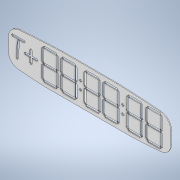
# Autodesk Inventor part: 7 Segment Clock
Saved by Autodesk Inventor 2021 (Build 250183000, 183)
## iProperties
Created: 2020-06-26
Part Number: 7 Segment Clock
Material: White
Document SubType Name: Modeling
Designer: dech3
Density: 1.188 g/cm^3
Appearance: Polycarbonate - Clear
Author: dech3
Autodesk Inventor part; units mm, degrees
(part 1 of 2)
ref_plane "YZ Plane" through (0, 0, 0) normal (1, 0, 0) x (0, 1, 0)
ref_plane "XZ Plane" through (0, 0, 0) normal (0, 1, 0) x (-1, 0, 0)
ref_plane "XY Plane" through (0, 0, 0) normal (0, 0, 1) x (1, 0, 0)
sketch "Single Segment" plane through (0, 0, 0) normal (0, 0, 1) x (1, 0, 0)
  arc A0 (130.9839, -3.9071) -> (131.691, -4.2) centre (131.691, -3.2) ccw
  arc A1 (131.691, 3.8) -> (130.9839, 3.5071) centre (131.691, 2.8) ccw
  line L0 (130.9839, -3.9071) -> (128.0768, -1)
  line L1 (130.9839, 3.5071) -> (128.0768, 0.6)
  line L2 (128.0768, -0.2) -> (128.0768, -1)
  line L3 (128.0768, -0.2) -> (128.0768, 0.6)
  line L4 (131.691, 3.8) -> (174.4626, 3.8)
  line L5 (174.4626, -4.2) -> (131.691, -4.2)
  arc A2 (175.1697, 3.5071) -> (174.4626, 3.8) centre (174.4626, 2.8) ccw
  line L6 (175.1697, 3.5071) -> (178.0768, 0.6)
  line L7 (178.0768, -0.2) -> (178.0768, 0.6)
  line L8 (178.0768, -0.2) -> (178.0768, -1)
  arc A3 (174.4626, -4.2) -> (175.1697, -3.9071) centre (174.4626, -3.2) ccw
  line L9 (175.1697, -3.9071) -> (178.0768, -1)
  point P0 (153.0768, 0)
  point P1 (131.2768, -4.2)
  point P2 (131.2768, 3.8)
  point P3 (174.8768, 3.8)
  point P4 (174.8768, -4.2)
  dimension "d105" = 3.2
  dimension "d108" = 3.2
  dimension "d111" = 3.2
  dimension "d112" = 3.2
  dimension "d113" = 3.2
  dimension "d114" = 3.2
  dimension "d115" = 3.2
  dimension "d116" = 1
  dimension "d117" = 8
  dimension "d118" = 8
  dimension "d121" = 3.2
  dimension "d122" = 3.2
  dimension "d123" = 50
  dimension "d126" = 135
  dimension "d127" = 50
  dimension "d128" = 135
  dimension "d129" = 4
  dimension "d130" = 4
  measures "d105" horizontal distance of point (131.277, -4.2) L0.end
  measures "d108" horizontal distance of L7.end point (174.877, 3.8)
  measures "d111" horizontal distance of point (131.277, 3.8) L3.end
  measures "d112" horizontal distance of L9.end point (174.877, -4.2)
  measures "d113" horizontal distance of L9.end point (174.877, -4.2)
  measures "d114" horizontal distance of point (131.277, 3.8) L3.end
  measures "d115" horizontal distance of point (131.277, -4.2) L0.end
  measures "d116" radius of A1
  measures "d117" distance of point (174.877, -4.2) point (174.877, 3.8)
  measures "d118" distance of point (131.277, -4.2) point (131.277, 3.8)
  measures "d121" horizontal distance of L7.end point (174.877, 3.8)
  measures "d122" horizontal distance of point (174.877, -4.2) L8.start
  measures "d123" distance of L8.start L3.start
  measures "d126" angle of L5 L9
  measures "d127" horizontal distance of L9.end L3.start
  measures "d128" angle of L4 L6
  measures "d129" vertical distance of L8.start point (174.877, -4.2)
  measures "d130" vertical distance of point (131.277, -4.2) L3.start
sketch "7 Segment Digit" plane through (0, 0, 0) normal (0, 0, 1) x (1, 0, 0)
  arc A0 (217.9071, 45.0929) -> (218.6142, 44.8) centre (218.6142, 45.8) ccw
  arc A1 (218.6142, 52.8) -> (217.9071, 52.5071) centre (218.6142, 51.8) ccw
  line L0 (217.9071, 45.0929) -> (215, 48)
  line L1 (217.9071, 52.5071) -> (215, 49.6)
  line L2 (215, 48.8) -> (215, 48)
  line L3 (215, 48.8) -> (215, 49.6)
  line L4 (218.6142, 52.8) -> (261.3858, 52.8)
  line L5 (261.3858, 44.8) -> (218.6142, 44.8)
  arc A2 (262.0929, 52.5071) -> (261.3858, 52.8) centre (261.3858, 51.8) ccw
  line L6 (262.0929, 52.5071) -> (265, 49.6)
  line L7 (265, 48.8) -> (265, 49.6)
  line L8 (265, 48.8) -> (265, 48)
  arc A3 (261.3858, 44.8) -> (262.0929, 45.0929) centre (261.3858, 45.8) ccw
  line L9 (262.0929, 45.0929) -> (265, 48)
  arc A4 (217.9071, -8.7071) -> (218.6142, -9) centre (218.6142, -8) ccw
  arc A5 (218.6142, -1) -> (217.9071, -1.2929) centre (218.6142, -2) ccw
  line L10 (217.9071, -8.7071) -> (215, -5.8)
  line L11 (217.9071, -1.2929) -> (215, -4.2)
  line L12 (215, -5) -> (215, -5.8)
  line L13 (215, -5) -> (215, -4.2)
  line L14 (218.6142, -1) -> (261.3858, -1)
  line L15 (261.3858, -9) -> (218.6142, -9)
  arc A6 (262.0929, -1.2929) -> (261.3858, -1) centre (261.3858, -2) ccw
  line L16 (262.0929, -1.2929) -> (265, -4.2)
  line L17 (265, -5) -> (265, -4.2)
  line L18 (265, -5) -> (265, -5.8)
  arc A7 (261.3858, -9) -> (262.0929, -8.7071) centre (261.3858, -8) ccw
  line L19 (262.0929, -8.7071) -> (265, -5.8)
  arc A8 (216.8071, -0.1929) -> (217.1, 0.5142) centre (216.1, 0.5142) ccw
  arc A9 (209.1, 0.5142) -> (209.3929, -0.1929) centre (210.1, 0.5142) ccw
  line L20 (216.8071, -0.1929) -> (213.9, -3.1)
  line L21 (209.3929, -0.1929) -> (212.3, -3.1)
  line L22 (213.1, -3.1) -> (213.9, -3.1)
  line L23 (213.1, -3.1) -> (212.3, -3.1)
  line L24 (209.1, 0.5142) -> (209.1, 43.2858)
  line L25 (217.1, 43.2858) -> (217.1, 0.5142)
  arc A10 (209.3929, 43.9929) -> (209.1, 43.2858) centre (210.1, 43.2858) ccw
  line L26 (209.3929, 43.9929) -> (212.3, 46.9)
  line L27 (213.1, 46.9) -> (212.3, 46.9)
  line L28 (213.1, 46.9) -> (213.9, 46.9)
  arc A11 (217.1, 43.2858) -> (216.8071, 43.9929) centre (216.1, 43.2858) ccw
  line L29 (216.8071, 43.9929) -> (213.9, 46.9)
  arc A12 (216.8071, -53.9929) -> (217.1, -53.2858) centre (216.1, -53.2858) ccw
  arc A13 (209.1, -53.2858) -> (209.3929, -53.9929) centre (210.1, -53.2858) ccw
  line L30 (216.8071, -53.9929) -> (213.9, -56.9)
  line L31 (209.3929, -53.9929) -> (212.3, -56.9)
  line L32 (213.1, -56.9) -> (213.9, -56.9)
  line L33 (213.1, -56.9) -> (212.3, -56.9)
  line L34 (209.1, -53.2858) -> (209.1, -10.5142)
  line L35 (217.1, -10.5142) -> (217.1, -53.2858)
  arc A14 (209.3929, -9.8071) -> (209.1, -10.5142) centre (210.1, -10.5142) ccw
  line L36 (209.3929, -9.8071) -> (212.3, -6.9)
  line L37 (213.1, -6.9) -> (212.3, -6.9)
  line L38 (213.1, -6.9) -> (213.9, -6.9)
  arc A15 (217.1, -10.5142) -> (216.8071, -9.8071) centre (216.1, -10.5142) ccw
  line L39 (216.8071, -9.8071) -> (213.9, -6.9)
  arc A16 (270.6071, -0.1929) -> (270.9, 0.5142) centre (269.9, 0.5142) ccw
  arc A17 (262.9, 0.5142) -> (263.1929, -0.1929) centre (263.9, 0.5142) ccw
  line L40 (270.6071, -0.1929) -> (267.7, -3.1)
  line L41 (263.1929, -0.1929) -> (266.1, -3.1)
  line L42 (266.9, -3.1) -> (267.7, -3.1)
  line L43 (266.9, -3.1) -> (266.1, -3.1)
  line L44 (262.9, 0.5142) -> (262.9, 43.2858)
  line L45 (270.9, 43.2858) -> (270.9, 0.5142)
  arc A18 (263.1929, 43.9929) -> (262.9, 43.2858) centre (263.9, 43.2858) ccw
  line L46 (263.1929, 43.9929) -> (266.1, 46.9)
  line L47 (266.9, 46.9) -> (266.1, 46.9)
  line L48 (266.9, 46.9) -> (267.7, 46.9)
  arc A19 (270.9, 43.2858) -> (270.6071, 43.9929) centre (269.9, 43.2858) ccw
  line L49 (270.6071, 43.9929) -> (267.7, 46.9)
  arc A20 (270.6071, -53.9929) -> (270.9, -53.2858) centre (269.9, -53.2858) ccw
  arc A21 (262.9, -53.2858) -> (263.1929, -53.9929) centre (263.9, -53.2858) ccw
  line L50 (270.6071, -53.9929) -> (267.7, -56.9)
  line L51 (263.1929, -53.9929) -> (266.1, -56.9)
  line L52 (266.9, -56.9) -> (267.7, -56.9)
  line L53 (266.9, -56.9) -> (266.1, -56.9)
  line L54 (262.9, -53.2858) -> (262.9, -10.5142)
  line L55 (270.9, -10.5142) -> (270.9, -53.2858)
  arc A22 (263.1929, -9.8071) -> (262.9, -10.5142) centre (263.9, -10.5142) ccw
  line L56 (263.1929, -9.8071) -> (266.1, -6.9)
  line L57 (266.9, -6.9) -> (266.1, -6.9)
  line L58 (266.9, -6.9) -> (267.7, -6.9)
  arc A23 (270.9, -10.5142) -> (270.6071, -9.8071) centre (269.9, -10.5142) ccw
  line L59 (270.6071, -9.8071) -> (267.7, -6.9)
  arc A24 (217.9071, -62.5071) -> (218.6142, -62.8) centre (218.6142, -61.8) ccw
  arc A25 (218.6142, -54.8) -> (217.9071, -55.0929) centre (218.6142, -55.8) ccw
  line L60 (217.9071, -62.5071) -> (215, -59.6)
  line L61 (217.9071, -55.0929) -> (215, -58)
  line L62 (215, -58.8) -> (215, -59.6)
  line L63 (215, -58.8) -> (215, -58)
  line L64 (218.6142, -54.8) -> (261.3858, -54.8)
  line L65 (261.3858, -62.8) -> (218.6142, -62.8)
  arc A26 (262.0929, -55.0929) -> (261.3858, -54.8) centre (261.3858, -55.8) ccw
  line L66 (262.0929, -55.0929) -> (265, -58)
  line L67 (265, -58.8) -> (265, -58)
  line L68 (265, -58.8) -> (265, -59.6)
  arc A27 (261.3858, -62.8) -> (262.0929, -62.5071) centre (261.3858, -61.8) ccw
  line L69 (262.0929, -62.5071) -> (265, -59.6)
  point P0 (239.8857, -4.9143)
  dimension "d131" = 1.1
  dimension "d132" = 1.1
  dimension "d137" = 1.1
  dimension "d138" = 1.1
  dimension "d139" = 1.1
  dimension "d140" = 1.1
  dimension "d141" = 1.1
  dimension "d142" = 1.1
  dimension "d143" = 1.1
  dimension "d144" = 1.1
  dimension "d145" = 1.1
  dimension "d146" = 1.1
  dimension "d150" = 1.1
  dimension "d151" = 1.1
  dimension "d152" = 1.1
  dimension "d153" = 1.1
sketch "Slanted Segment Large" plane through (0, 0, 0) normal (0, 0, 1) x (1, 0, 0)
  line L0 (-252.8296, -124.6537) -> (-254.4296, -124.6537)
  line L1 (-254.4296, -124.6537) -> (-257.6296, -127.8537)
  line L2 (-257.6296, -127.8537) -> (-261.6917, -184.8537)
  line L3 (-253.6917, -184.8537) -> (-249.6296, -127.8537)
  line L4 (-249.6296, -127.8537) -> (-252.8296, -124.6537)
  line L5 (-261.6917, -184.8537) -> (-258.4917, -188.0537)
  line L6 (-258.4917, -188.0537) -> (-256.8917, -188.0537)
  line L7 (-256.8917, -188.0537) -> (-253.6917, -184.8537)
  point P0 (-253.3255, -154.094)
  point P1 (-253.6296, -124.6537)
  dimension "d294" = 3.2
  dimension "d295" = 3.2
  dimension "d296" = 8
  dimension "d297" = 3.2
  dimension "d298" = 3.2
  dimension "d299" = 57
  dimension "d304" = 3.2
  dimension "d305" = 3.2
  dimension "d306" = 3.2
  dimension "d307" = 3.2
  measures "d294" horizontal distance of L0.end L1.end
  measures "d295" horizontal distance of L3.end L0.start
  measures "d296" distance of L3.end L1.end
  measures "d297" horizontal distance of L3.end L0.start
  measures "d298" horizontal distance of L0.end L1.end
  measures "d299" vertical distance of L3.end L3.start
  measures "d304" horizontal distance of L5.end L2.end
  measures "d305" horizontal distance of L3.start L6.end
  measures "d306" horizontal distance of L2.end L5.end
  measures "d307" horizontal distance of L3.start L6.end
sketch "+ sign" plane through (0, 0, 0) normal (0, 0, 1) x (1, 0, 0)
  line L0 (-226.2607, 18.0992) -> (-229.1679, 15.1921)
  line L1 (-229.4607, 14.485) -> (-229.4607, -2.7008)
  line L2 (-246.6465, -2.7008) -> (-229.4607, -2.7008)
  line L3 (-247.3536, -2.9937) -> (-250.2607, -5.9008)
  line L4 (-250.2607, -5.9008) -> (-250.2607, -7.5008)
  line L5 (-246.6465, -10.7008) -> (-229.4607, -10.7008)
  line L6 (-229.4607, -10.7008) -> (-229.4607, -27.8865)
  line L7 (-226.2607, -31.5008) -> (-224.6607, -31.5008)
  line L8 (-224.6607, -31.5008) -> (-221.7536, -28.5937)
  line L9 (-221.4607, -27.8865) -> (-221.4607, -10.7008)
  line L10 (-204.275, -2.7008) -> (-221.4607, -2.7008)
  line L11 (-204.275, -10.7008) -> (-221.4607, -10.7008)
  line L12 (-203.5679, -2.9937) -> (-200.6607, -5.9008)
  line L13 (-200.6607, -5.9008) -> (-200.6607, -7.5008)
  line L14 (-247.3536, -10.4079) -> (-250.2607, -7.5008)
  line L15 (-229.1679, -28.5937) -> (-226.2607, -31.5008)
  line L16 (-203.5679, -10.4079) -> (-200.6607, -7.5008)
  line L17 (-221.4607, -2.7008) -> (-221.4607, 14.485)
  line L18 (-221.7536, 15.1921) -> (-224.6607, 18.0992)
  line L19 (-224.6607, 18.0992) -> (-226.2607, 18.0992)
  arc A0 (-229.1679, 15.1921) -> (-229.4607, 14.485) centre (-228.4607, 14.485) ccw
  arc A1 (-221.4607, 14.485) -> (-221.7536, 15.1921) centre (-222.4607, 14.485) ccw
  arc A2 (-203.5679, -2.9937) -> (-204.275, -2.7008) centre (-204.275, -3.7008) ccw
  arc A3 (-204.275, -10.7008) -> (-203.5679, -10.4079) centre (-204.275, -9.7008) ccw
  arc A4 (-229.4607, -27.8865) -> (-229.1679, -28.5937) centre (-228.4607, -27.8865) ccw
  arc A5 (-221.7536, -28.5937) -> (-221.4607, -27.8865) centre (-222.4607, -27.8865) ccw
  arc A6 (-247.3536, -10.4079) -> (-246.6465, -10.7008) centre (-246.6465, -9.7008) ccw
  arc A7 (-246.6465, -2.7008) -> (-247.3536, -2.9937) centre (-246.6465, -3.7008) ccw
  point P0 (-225.4266, -6.7349)
  point P1 (-229.4607, 14.8992)
  point P2 (-247.0607, -2.7008)
  point P3 (-247.0607, -10.7008)
  point P4 (-229.4607, -28.3008)
  point P5 (-221.4607, -28.3008)
  point P6 (-203.8607, -2.7008)
  point P7 (-203.8607, -10.7008)
  point P8 (-221.4607, 14.8992)
  dimension "d259" = 3.2
  dimension "d260" = 3.2
  dimension "d261" = 3.2
  dimension "d262" = 3.2
  dimension "d263" = 3.2
  dimension "d264" = 3.2
  dimension "d265" = 3.2
  dimension "d266" = 3.2
  dimension "d267" = 3.2
  dimension "d268" = 3.2
  dimension "d269" = 3.2
  dimension "d270" = 3.2
  dimension "d271" = 3.2
  dimension "d272" = 0
  dimension "d273" = 0
  dimension "d274" = 8
  dimension "d275" = 8
  dimension "d276" = 0
  dimension "d277" = 0
  dimension "d278" = 3.2
  dimension "d279" = 3.2
  dimension "d280" = 3.2
  dimension "d281" = 90
  dimension "d284" = 17.6
  dimension "d285" = 17.6
  dimension "d286" = 17.6
  dimension "d287" = 17.6
  dimension "d288" = 17.6
  dimension "d289" = 0
  dimension "d290" = 17.6
  dimension "d292" = 1
  dimension "d293" = 1
  measures "d259" distance from line of point (-247.061, -2.701) L4
  measures "d260" horizontal distance of point (-247.061, -2.701) L3.end
  measures "d261" horizontal distance of point (-247.061, -10.701) L14.end
  measures "d262" horizontal distance of point (-247.061, -10.701) L14.end
  measures "d263" horizontal distance of L15.end point (-229.461, -28.301)
  measures "d264" horizontal distance of point (-229.461, -28.301) L15.end
  measures "d265" horizontal distance of point (-221.461, -28.301) L7.end
  measures "d266" horizontal distance of L7.end point (-221.461, -28.301)
  measures "d267" horizontal distance of L16.end point (-203.861, -10.701)
  measures "d268" horizontal distance of point (-203.861, -10.701) L16.end
  measures "d269" horizontal distance of point (-203.861, -2.701) L12.end
  measures "d270" horizontal distance of point (-203.861, -2.701) L12.end
  measures "d271" horizontal distance of L18.end point (-221.461, 14.899)
  measures "d272" distance between parallel lines of L17 L9
  measures "d273" distance between parallel lines of L1 L6
  measures "d274" distance between parallel lines of L17 L1
  measures "d275" distance between parallel lines of L5 L2
  measures "d276" distance between parallel lines of L2 L10
  measures "d277" distance between parallel lines of L5 L11
  measures "d278" horizontal distance of L19.end point (-229.461, 14.899)
  measures "d279" horizontal distance of L19.end point (-229.461, 14.899)
  measures "d280" horizontal distance of L18.end point (-221.461, 14.899)
  measures "d281" angle of L10 L17
  measures "d284" distance of L1.end point (-247.061, -2.701)
  measures "d285" distance of point (-203.861, -2.701) L17.start
  measures "d286" distance of point (-221.461, 14.899) L17.start
  measures "d287" distance of point (-221.461, -28.301) L9.end
  measures "d288" distance of point (-229.461, -28.301) L5.end
  measures "d289" distance of L9.end L11.end
  measures "d290" distance of L9.end point (-203.861, -10.701)
  measures "d292" radius of A0
  measures "d293" radius of A4
sketch "Dot" plane through (0, 0, 0) normal (0, 0, 1) x (1, 0, 0)
  line L0 (-34.9663, 29.5091) -> (-32.9663, 29.5091)
  line L1 (-32.9663, 29.5091) -> (-29.7663, 26.3091)
  line L2 (-29.7663, 26.3091) -> (-29.7663, 24.3091)
  line L3 (-29.7663, 24.3091) -> (-32.9663, 21.1091)
  line L4 (-32.9663, 21.1091) -> (-34.9663, 21.1091)
  line L5 (-34.9663, 21.1091) -> (-38.1663, 24.3091)
  line L6 (-38.1663, 24.3091) -> (-38.1663, 26.3091)
  line L7 (-38.1663, 26.3091) -> (-34.9663, 29.5091)
  point P0 (-33.9663, 25.3091)
  dimension "d311" = 3.2
  dimension "d312" = 3.2
  dimension "d314" = 3.2
  dimension "d315" = 3.2
  dimension "d316" = 3.2
  dimension "d317" = 3.2
  dimension "d318" = 3.2
  dimension "d319" = 3.2
  dimension "d320" = 2
  dimension "d321" = 2
  dimension "d322" = 2
  dimension "d323" = 2
  measures "d311" horizontal distance of L1.end L0.end
  measures "d312" horizontal distance of L0.start L6.end
  measures "d314" horizontal distance of L0.start L6.end
  measures "d315" horizontal distance of L1.end L0.end
  measures "d316" horizontal distance of L4.end L5.end
  measures "d317" horizontal distance of L2.end L3.end
  measures "d318" horizontal distance of L2.end L3.end
  measures "d319" horizontal distance of L5.end L4.end
  measures "d320" distance of L1.end L2.end
  measures "d321" distance of L0.end L0.start
  measures "d322" distance of L3.end L4.end
  measures "d323" distance of L6.end L5.end
sketch "Clock Face with T +-" plane through (0, 0, 0) normal (0, 0, 1) x (1, 0, 0)
  arc A0 (144.2071, 46.2929) -> (144.9142, 46) centre (144.9142, 47) ccw
  arc A1 (144.9142, 54) -> (144.2071, 53.7071) centre (144.9142, 53) ccw
  line L0 (144.2071, 46.2929) -> (141.3, 49.2)
  line L1 (144.2071, 53.7071) -> (141.3, 50.8)
  line L2 (141.3, 50) -> (141.3, 49.2)
  line L3 (141.3, 50) -> (141.3, 50.8)
  line L4 (144.9142, 54) -> (187.6858, 54)
  line L5 (187.6858, 46) -> (144.9142, 46)
  arc A2 (188.3929, 53.7071) -> (187.6858, 54) centre (187.6858, 53) ccw
  line L6 (188.3929, 53.7071) -> (191.3, 50.8)
  line L7 (191.3, 50) -> (191.3, 50.8)
  line L8 (191.3, 50) -> (191.3, 49.2)
  arc A3 (187.6858, 46) -> (188.3929, 46.2929) centre (187.6858, 47) ccw
  line L9 (188.3929, 46.2929) -> (191.3, 49.2)
  arc A4 (144.2071, -7.5071) -> (144.9142, -7.8) centre (144.9142, -6.8) ccw
  arc A5 (144.9142, 0.2) -> (144.2071, -0.0929) centre (144.9142, -0.8) ccw
  line L10 (144.2071, -7.5071) -> (141.3, -4.6)
  line L11 (144.2071, -0.0929) -> (141.3, -3)
  line L12 (141.3, -3.8) -> (141.3, -4.6)
  line L13 (141.3, -3.8) -> (141.3, -3)
  line L14 (144.9142, 0.2) -> (187.6858, 0.2)
  line L15 (187.6858, -7.8) -> (144.9142, -7.8)
  arc A6 (188.3929, -0.0929) -> (187.6858, 0.2) centre (187.6858, -0.8) ccw
  line L16 (188.3929, -0.0929) -> (191.3, -3)
  line L17 (191.3, -3.8) -> (191.3, -3)
  line L18 (191.3, -3.8) -> (191.3, -4.6)
  arc A7 (187.6858, -7.8) -> (188.3929, -7.5071) centre (187.6858, -6.8) ccw
  line L19 (188.3929, -7.5071) -> (191.3, -4.6)
  arc A8 (143.1071, 1.0071) -> (143.4, 1.7142) centre (142.4, 1.7142) ccw
  arc A9 (135.4, 1.7142) -> (135.6929, 1.0071) centre (136.4, 1.7142) ccw
  line L20 (143.1071, 1.0071) -> (140.2, -1.9)
  line L21 (135.6929, 1.0071) -> (138.6, -1.9)
  line L22 (139.4, -1.9) -> (140.2, -1.9)
  line L23 (139.4, -1.9) -> (138.6, -1.9)
  line L24 (135.4, 1.7142) -> (135.4, 44.4858)
  line L25 (143.4, 44.4858) -> (143.4, 1.7142)
  arc A10 (135.6929, 45.1929) -> (135.4, 44.4858) centre (136.4, 44.4858) ccw
  line L26 (135.6929, 45.1929) -> (138.6, 48.1)
  line L27 (139.4, 48.1) -> (138.6, 48.1)
  line L28 (139.4, 48.1) -> (140.2, 48.1)
  arc A11 (143.4, 44.4858) -> (143.1071, 45.1929) centre (142.4, 44.4858) ccw
  line L29 (143.1071, 45.1929) -> (140.2, 48.1)
  arc A12 (143.1071, -52.7929) -> (143.4, -52.0858) centre (142.4, -52.0858) ccw
  arc A13 (135.4, -52.0858) -> (135.6929, -52.7929) centre (136.4, -52.0858) ccw
  line L30 (143.1071, -52.7929) -> (140.2, -55.7)
  line L31 (135.6929, -52.7929) -> (138.6, -55.7)
  line L32 (139.4, -55.7) -> (140.2, -55.7)
  line L33 (139.4, -55.7) -> (138.6, -55.7)
  line L34 (135.4, -52.0858) -> (135.4, -9.3142)
  line L35 (143.4, -9.3142) -> (143.4, -52.0858)
  arc A14 (135.6929, -8.6071) -> (135.4, -9.3142) centre (136.4, -9.3142) ccw
  line L36 (135.6929, -8.6071) -> (138.6, -5.7)
  line L37 (139.4, -5.7) -> (138.6, -5.7)
  line L38 (139.4, -5.7) -> (140.2, -5.7)
  arc A15 (143.4, -9.3142) -> (143.1071, -8.6071) centre (142.4, -9.3142) ccw
  line L39 (143.1071, -8.6071) -> (140.2, -5.7)
  arc A16 (196.9071, 1.0071) -> (197.2, 1.7142) centre (196.2, 1.7142) ccw
  arc A17 (189.2, 1.7142) -> (189.4929, 1.0071) centre (190.2, 1.7142) ccw
  line L40 (196.9071, 1.0071) -> (194, -1.9)
  line L41 (189.4929, 1.0071) -> (192.4, -1.9)
  line L42 (193.2, -1.9) -> (194, -1.9)
  line L43 (193.2, -1.9) -> (192.4, -1.9)
  line L44 (189.2, 1.7142) -> (189.2, 44.4858)
  line L45 (197.2, 44.4858) -> (197.2, 1.7142)
  arc A18 (189.4929, 45.1929) -> (189.2, 44.4858) centre (190.2, 44.4858) ccw
  line L46 (189.4929, 45.1929) -> (192.4, 48.1)
  line L47 (193.2, 48.1) -> (192.4, 48.1)
  line L48 (193.2, 48.1) -> (194, 48.1)
  arc A19 (197.2, 44.4858) -> (196.9071, 45.1929) centre (196.2, 44.4858) ccw
  line L49 (196.9071, 45.1929) -> (194, 48.1)
  arc A20 (196.9071, -52.7929) -> (197.2, -52.0858) centre (196.2, -52.0858) ccw
  arc A21 (189.2, -52.0858) -> (189.4929, -52.7929) centre (190.2, -52.0858) ccw
  line L50 (196.9071, -52.7929) -> (194, -55.7)
  line L51 (189.4929, -52.7929) -> (192.4, -55.7)
  line L52 (193.2, -55.7) -> (194, -55.7)
  line L53 (193.2, -55.7) -> (192.4, -55.7)
  line L54 (189.2, -52.0858) -> (189.2, -9.3142)
  line L55 (197.2, -9.3142) -> (197.2, -52.0858)
  arc A22 (189.4929, -8.6071) -> (189.2, -9.3142) centre (190.2, -9.3142) ccw
  line L56 (189.4929, -8.6071) -> (192.4, -5.7)
  line L57 (193.2, -5.7) -> (192.4, -5.7)
  line L58 (193.2, -5.7) -> (194, -5.7)
  arc A23 (197.2, -9.3142) -> (196.9071, -8.6071) centre (196.2, -9.3142) ccw
  line L59 (196.9071, -8.6071) -> (194, -5.7)
  arc A24 (144.2071, -61.3071) -> (144.9142, -61.6) centre (144.9142, -60.6) ccw
  arc A25 (144.9142, -53.6) -> (144.2071, -53.8929) centre (144.9142, -54.6) ccw
  line L60 (144.2071, -61.3071) -> (141.3, -58.4)
  line L61 (144.2071, -53.8929) -> (141.3, -56.8)
  line L62 (141.3, -57.6) -> (141.3, -58.4)
  line L63 (141.3, -57.6) -> (141.3, -56.8)
  line L64 (144.9142, -53.6) -> (187.6858, -53.6)
  line L65 (187.6858, -61.6) -> (144.9142, -61.6)
  arc A26 (188.3929, -53.8929) -> (187.6858, -53.6) centre (187.6858, -54.6) ccw
  line L66 (188.3929, -53.8929) -> (191.3, -56.8)
  line L67 (191.3, -57.6) -> (191.3, -56.8)
  line L68 (191.3, -57.6) -> (191.3, -58.4)
  arc A27 (187.6858, -61.6) -> (188.3929, -61.3071) centre (187.6858, -60.6) ccw
  line L69 (188.3929, -61.3071) -> (191.3, -58.4)
  arc A28 (57.4071, 46.2929) -> (58.1142, 46) centre (58.1142, 47) ccw
  arc A29 (58.1142, 54) -> (57.4071, 53.7071) centre (58.1142, 53) ccw
  line L70 (57.4071, 46.2929) -> (54.5, 49.2)
  line L71 (57.4071, 53.7071) -> (54.5, 50.8)
  line L72 (54.5, 50) -> (54.5, 49.2)
  line L73 (54.5, 50) -> (54.5, 50.8)
  line L74 (58.1142, 54) -> (100.8858, 54)
  line L75 (100.8858, 46) -> (58.1142, 46)
  arc A30 (101.5929, 53.7071) -> (100.8858, 54) centre (100.8858, 53) ccw
  line L76 (101.5929, 53.7071) -> (104.5, 50.8)
  line L77 (104.5, 50) -> (104.5, 50.8)
  line L78 (104.5, 50) -> (104.5, 49.2)
  arc A31 (100.8858, 46) -> (101.5929, 46.2929) centre (100.8858, 47) ccw
  line L79 (101.5929, 46.2929) -> (104.5, 49.2)
  arc A32 (57.4071, -7.5071) -> (58.1142, -7.8) centre (58.1142, -6.8) ccw
  arc A33 (58.1142, 0.2) -> (57.4071, -0.0929) centre (58.1142, -0.8) ccw
  line L80 (57.4071, -7.5071) -> (54.5, -4.6)
  line L81 (57.4071, -0.0929) -> (54.5, -3)
  line L82 (54.5, -3.8) -> (54.5, -4.6)
  line L83 (54.5, -3.8) -> (54.5, -3)
  line L84 (58.1142, 0.2) -> (100.8858, 0.2)
  line L85 (100.8858, -7.8) -> (58.1142, -7.8)
  arc A34 (101.5929, -0.0929) -> (100.8858, 0.2) centre (100.8858, -0.8) ccw
  line L86 (101.5929, -0.0929) -> (104.5, -3)
  line L87 (104.5, -3.8) -> (104.5, -3)
  line L88 (104.5, -3.8) -> (104.5, -4.6)
  arc A35 (100.8858, -7.8) -> (101.5929, -7.5071) centre (100.8858, -6.8) ccw
  line L89 (101.5929, -7.5071) -> (104.5, -4.6)
  arc A36 (56.3071, 1.0071) -> (56.6, 1.7142) centre (55.6, 1.7142) ccw
  arc A37 (48.6, 1.7142) -> (48.8929, 1.0071) centre (49.6, 1.7142) ccw
  line L90 (56.3071, 1.0071) -> (53.4, -1.9)
  line L91 (48.8929, 1.0071) -> (51.8, -1.9)
  line L92 (52.6, -1.9) -> (53.4, -1.9)
  line L93 (52.6, -1.9) -> (51.8, -1.9)
  line L94 (48.6, 1.7142) -> (48.6, 44.4858)
  line L95 (56.6, 44.4858) -> (56.6, 1.7142)
  arc A38 (48.8929, 45.1929) -> (48.6, 44.4858) centre (49.6, 44.4858) ccw
  line L96 (48.8929, 45.1929) -> (51.8, 48.1)
  line L97 (52.6, 48.1) -> (51.8, 48.1)
  line L98 (52.6, 48.1) -> (53.4, 48.1)
  arc A39 (56.6, 44.4858) -> (56.3071, 45.1929) centre (55.6, 44.4858) ccw
  line L99 (56.3071, 45.1929) -> (53.4, 48.1)
  arc A40 (56.3071, -52.7929) -> (56.6, -52.0858) centre (55.6, -52.0858) ccw
  arc A41 (48.6, -52.0858) -> (48.8929, -52.7929) centre (49.6, -52.0858) ccw
  line L100 (56.3071, -52.7929) -> (53.4, -55.7)
  line L101 (48.8929, -52.7929) -> (51.8, -55.7)
  line L102 (52.6, -55.7) -> (53.4, -55.7)
  line L103 (52.6, -55.7) -> (51.8, -55.7)
  line L104 (48.6, -52.0858) -> (48.6, -9.3142)
  line L105 (56.6, -9.3142) -> (56.6, -52.0858)
  arc A42 (48.8929, -8.6071) -> (48.6, -9.3142) centre (49.6, -9.3142) ccw
  line L106 (48.8929, -8.6071) -> (51.8, -5.7)
  line L107 (52.6, -5.7) -> (51.8, -5.7)
  line L108 (52.6, -5.7) -> (53.4, -5.7)
  arc A43 (56.6, -9.3142) -> (56.3071, -8.6071) centre (55.6, -9.3142) ccw
  line L109 (56.3071, -8.6071) -> (53.4, -5.7)
  arc A44 (110.1071, 1.0071) -> (110.4, 1.7142) centre (109.4, 1.7142) ccw
  arc A45 (102.4, 1.7142) -> (102.6929, 1.0071) centre (103.4, 1.7142) ccw
  line L110 (110.1071, 1.0071) -> (107.2, -1.9)
  line L111 (102.6929, 1.0071) -> (105.6, -1.9)
  line L112 (106.4, -1.9) -> (107.2, -1.9)
  line L113 (106.4, -1.9) -> (105.6, -1.9)
  line L114 (102.4, 1.7142) -> (102.4, 44.4858)
  line L115 (110.4, 44.4858) -> (110.4, 1.7142)
  arc A46 (102.6929, 45.1929) -> (102.4, 44.4858) centre (103.4, 44.4858) ccw
  line L116 (102.6929, 45.1929) -> (105.6, 48.1)
  line L117 (106.4, 48.1) -> (105.6, 48.1)
  line L118 (106.4, 48.1) -> (107.2, 48.1)
  arc A47 (110.4, 44.4858) -> (110.1071, 45.1929) centre (109.4, 44.4858) ccw
  line L119 (110.1071, 45.1929) -> (107.2, 48.1)
  arc A48 (110.1071, -52.7929) -> (110.4, -52.0858) centre (109.4, -52.0858) ccw
  arc A49 (102.4, -52.0858) -> (102.6929, -52.7929) centre (103.4, -52.0858) ccw
  line L120 (110.1071, -52.7929) -> (107.2, -55.7)
  line L121 (102.6929, -52.7929) -> (105.6, -55.7)
  line L122 (106.4, -55.7) -> (107.2, -55.7)
  line L123 (106.4, -55.7) -> (105.6, -55.7)
  line L124 (102.4, -52.0858) -> (102.4, -9.3142)
  line L125 (110.4, -9.3142) -> (110.4, -52.0858)
  arc A50 (102.6929, -8.6071) -> (102.4, -9.3142) centre (103.4, -9.3142) ccw
  line L126 (102.6929, -8.6071) -> (105.6, -5.7)
  line L127 (106.4, -5.7) -> (105.6, -5.7)
  line L128 (106.4, -5.7) -> (107.2, -5.7)
  arc A51 (110.4, -9.3142) -> (110.1071, -8.6071) centre (109.4, -9.3142) ccw
  line L129 (110.1071, -8.6071) -> (107.2, -5.7)
  arc A52 (57.4071, -61.3071) -> (58.1142, -61.6) centre (58.1142, -60.6) ccw
  arc A53 (58.1142, -53.6) -> (57.4071, -53.8929) centre (58.1142, -54.6) ccw
  line L130 (57.4071, -61.3071) -> (54.5, -58.4)
  line L131 (57.4071, -53.8929) -> (54.5, -56.8)
  line L132 (54.5, -57.6) -> (54.5, -58.4)
  line L133 (54.5, -57.6) -> (54.5, -56.8)
  line L134 (58.1142, -53.6) -> (100.8858, -53.6)
  line L135 (100.8858, -61.6) -> (58.1142, -61.6)
  arc A54 (101.5929, -53.8929) -> (100.8858, -53.6) centre (100.8858, -54.6) ccw
  line L136 (101.5929, -53.8929) -> (104.5, -56.8)
  line L137 (104.5, -57.6) -> (104.5, -56.8)
  line L138 (104.5, -57.6) -> (104.5, -58.4)
  arc A55 (100.8858, -61.6) -> (101.5929, -61.3071) centre (100.8858, -60.6) ccw
  line L139 (101.5929, -61.3071) -> (104.5, -58.4)
  arc A56 (-11.8929, 46.2929) -> (-11.1858, 46) centre (-11.1858, 47) ccw
  arc A57 (-11.1858, 54) -> (-11.8929, 53.7071) centre (-11.1858, 53) ccw
  line L140 (-11.8929, 46.2929) -> (-14.8, 49.2)
  line L141 (-11.8929, 53.7071) -> (-14.8, 50.8)
  line L142 (-14.8, 50) -> (-14.8, 49.2)
  line L143 (-14.8, 50) -> (-14.8, 50.8)
  line L144 (-11.1858, 54) -> (31.5858, 54)
  line L145 (31.5858, 46) -> (-11.1858, 46)
  arc A58 (32.2929, 53.7071) -> (31.5858, 54) centre (31.5858, 53) ccw
  line L146 (32.2929, 53.7071) -> (35.2, 50.8)
  line L147 (35.2, 50) -> (35.2, 50.8)
  line L148 (35.2, 50) -> (35.2, 49.2)
  arc A59 (31.5858, 46) -> (32.2929, 46.2929) centre (31.5858, 47) ccw
  line L149 (32.2929, 46.2929) -> (35.2, 49.2)
  arc A60 (-11.8929, -7.5071) -> (-11.1858, -7.8) centre (-11.1858, -6.8) ccw
  arc A61 (-11.1858, 0.2) -> (-11.8929, -0.0929) centre (-11.1858, -0.8) ccw
  line L150 (-11.8929, -7.5071) -> (-14.8, -4.6)
  line L151 (-11.8929, -0.0929) -> (-14.8, -3)
  line L152 (-14.8, -3.8) -> (-14.8, -4.6)
  line L153 (-14.8, -3.8) -> (-14.8, -3)
  line L154 (-11.1858, 0.2) -> (31.5858, 0.2)
  line L155 (31.5858, -7.8) -> (-11.1858, -7.8)
  arc A62 (32.2929, -0.0929) -> (31.5858, 0.2) centre (31.5858, -0.8) ccw
  line L156 (32.2929, -0.0929) -> (35.2, -3)
  line L157 (35.2, -3.8) -> (35.2, -3)
  line L158 (35.2, -3.8) -> (35.2, -4.6)
  arc A63 (31.5858, -7.8) -> (32.2929, -7.5071) centre (31.5858, -6.8) ccw
  line L159 (32.2929, -7.5071) -> (35.2, -4.6)
  arc A64 (-12.9929, 1.0071) -> (-12.7, 1.7142) centre (-13.7, 1.7142) ccw
  arc A65 (-20.7, 1.7142) -> (-20.4071, 1.0071) centre (-19.7, 1.7142) ccw
  line L160 (-12.9929, 1.0071) -> (-15.9, -1.9)
  line L161 (-20.4071, 1.0071) -> (-17.5, -1.9)
  line L162 (-16.7, -1.9) -> (-15.9, -1.9)
  line L163 (-16.7, -1.9) -> (-17.5, -1.9)
  line L164 (-20.7, 1.7142) -> (-20.7, 44.4858)
  line L165 (-12.7, 44.4858) -> (-12.7, 1.7142)
  arc A66 (-20.4071, 45.1929) -> (-20.7, 44.4858) centre (-19.7, 44.4858) ccw
  line L166 (-20.4071, 45.1929) -> (-17.5, 48.1)
  line L167 (-16.7, 48.1) -> (-17.5, 48.1)
  line L168 (-16.7, 48.1) -> (-15.9, 48.1)
  arc A67 (-12.7, 44.4858) -> (-12.9929, 45.1929) centre (-13.7, 44.4858) ccw
  line L169 (-12.9929, 45.1929) -> (-15.9, 48.1)
  arc A68 (-12.9929, -52.7929) -> (-12.7, -52.0858) centre (-13.7, -52.0858) ccw
  arc A69 (-20.7, -52.0858) -> (-20.4071, -52.7929) centre (-19.7, -52.0858) ccw
  line L170 (-12.9929, -52.7929) -> (-15.9, -55.7)
  line L171 (-20.4071, -52.7929) -> (-17.5, -55.7)
  line L172 (-16.7, -55.7) -> (-15.9, -55.7)
  line L173 (-16.7, -55.7) -> (-17.5, -55.7)
  line L174 (-20.7, -52.0858) -> (-20.7, -9.3142)
  line L175 (-12.7, -9.3142) -> (-12.7, -52.0858)
  arc A70 (-20.4071, -8.6071) -> (-20.7, -9.3142) centre (-19.7, -9.3142) ccw
  line L176 (-20.4071, -8.6071) -> (-17.5, -5.7)
  line L177 (-16.7, -5.7) -> (-17.5, -5.7)
  line L178 (-16.7, -5.7) -> (-15.9, -5.7)
  arc A71 (-12.7, -9.3142) -> (-12.9929, -8.6071) centre (-13.7, -9.3142) ccw
  line L179 (-12.9929, -8.6071) -> (-15.9, -5.7)
  arc A72 (40.8071, 1.0071) -> (41.1, 1.7142) centre (40.1, 1.7142) ccw
  arc A73 (33.1, 1.7142) -> (33.3929, 1.0071) centre (34.1, 1.7142) ccw
  line L180 (40.8071, 1.0071) -> (37.9, -1.9)
  line L181 (33.3929, 1.0071) -> (36.3, -1.9)
  line L182 (37.1, -1.9) -> (37.9, -1.9)
  line L183 (37.1, -1.9) -> (36.3, -1.9)
  line L184 (33.1, 1.7142) -> (33.1, 44.4858)
  line L185 (41.1, 44.4858) -> (41.1, 1.7142)
  arc A74 (33.3929, 45.1929) -> (33.1, 44.4858) centre (34.1, 44.4858) ccw
  line L186 (33.3929, 45.1929) -> (36.3, 48.1)
  line L187 (37.1, 48.1) -> (36.3, 48.1)
  line L188 (37.1, 48.1) -> (37.9, 48.1)
  arc A75 (41.1, 44.4858) -> (40.8071, 45.1929) centre (40.1, 44.4858) ccw
  line L189 (40.8071, 45.1929) -> (37.9, 48.1)
  arc A76 (40.8071, -52.7929) -> (41.1, -52.0858) centre (40.1, -52.0858) ccw
  arc A77 (33.1, -52.0858) -> (33.3929, -52.7929) centre (34.1, -52.0858) ccw
  line L190 (40.8071, -52.7929) -> (37.9, -55.7)
  line L191 (33.3929, -52.7929) -> (36.3, -55.7)
  line L192 (37.1, -55.7) -> (37.9, -55.7)
  line L193 (37.1, -55.7) -> (36.3, -55.7)
  line L194 (33.1, -52.0858) -> (33.1, -9.3142)
  line L195 (41.1, -9.3142) -> (41.1, -52.0858)
  arc A78 (33.3929, -8.6071) -> (33.1, -9.3142) centre (34.1, -9.3142) ccw
  line L196 (33.3929, -8.6071) -> (36.3, -5.7)
  line L197 (37.1, -5.7) -> (36.3, -5.7)
  line L198 (37.1, -5.7) -> (37.9, -5.7)
  arc A79 (41.1, -9.3142) -> (40.8071, -8.6071) centre (40.1, -9.3142) ccw
  line L199 (40.8071, -8.6071) -> (37.9, -5.7)
  arc A80 (-11.8929, -61.3071) -> (-11.1858, -61.6) centre (-11.1858, -60.6) ccw
  arc A81 (-11.1858, -53.6) -> (-11.8929, -53.8929) centre (-11.1858, -54.6) ccw
  line L200 (-11.8929, -61.3071) -> (-14.8, -58.4)
  line L201 (-11.8929, -53.8929) -> (-14.8, -56.8)
  line L202 (-14.8, -57.6) -> (-14.8, -58.4)
  line L203 (-14.8, -57.6) -> (-14.8, -56.8)
  line L204 (-11.1858, -53.6) -> (31.5858, -53.6)
  line L205 (31.5858, -61.6) -> (-11.1858, -61.6)
  arc A82 (32.2929, -53.8929) -> (31.5858, -53.6) centre (31.5858, -54.6) ccw
  line L206 (32.2929, -53.8929) -> (35.2, -56.8)
  line L207 (35.2, -57.6) -> (35.2, -56.8)
  line L208 (35.2, -57.6) -> (35.2, -58.4)
  arc A83 (31.5858, -61.6) -> (32.2929, -61.3071) centre (31.5858, -60.6) ccw
  line L209 (32.2929, -61.3071) -> (35.2, -58.4)
  arc A84 (-98.6929, 46.2929) -> (-97.9858, 46) centre (-97.9858, 47) ccw
  arc A85 (-97.9858, 54) -> (-98.6929, 53.7071) centre (-97.9858, 53) ccw
  line L210 (-98.6929, 46.2929) -> (-101.6, 49.2)
  line L211 (-98.6929, 53.7071) -> (-101.6, 50.8)
  line L212 (-101.6, 50) -> (-101.6, 49.2)
  line L213 (-101.6, 50) -> (-101.6, 50.8)
  line L214 (-97.9858, 54) -> (-55.2142, 54)
  line L215 (-55.2142, 46) -> (-97.9858, 46)
  arc A86 (-54.5071, 53.7071) -> (-55.2142, 54) centre (-55.2142, 53) ccw
  line L216 (-54.5071, 53.7071) -> (-51.6, 50.8)
  line L217 (-51.6, 50) -> (-51.6, 50.8)
  line L218 (-51.6, 50) -> (-51.6, 49.2)
  arc A87 (-55.2142, 46) -> (-54.5071, 46.2929) centre (-55.2142, 47) ccw
  line L219 (-54.5071, 46.2929) -> (-51.6, 49.2)
  arc A88 (-98.6929, -7.5071) -> (-97.9858, -7.8) centre (-97.9858, -6.8) ccw
  arc A89 (-97.9858, 0.2) -> (-98.6929, -0.0929) centre (-97.9858, -0.8) ccw
  line L220 (-98.6929, -7.5071) -> (-101.6, -4.6)
  line L221 (-98.6929, -0.0929) -> (-101.6, -3)
  line L222 (-101.6, -3.8) -> (-101.6, -4.6)
  line L223 (-101.6, -3.8) -> (-101.6, -3)
  line L224 (-97.9858, 0.2) -> (-55.2142, 0.2)
  line L225 (-55.2142, -7.8) -> (-97.9858, -7.8)
  arc A90 (-54.5071, -0.0929) -> (-55.2142, 0.2) centre (-55.2142, -0.8) ccw
  line L226 (-54.5071, -0.0929) -> (-51.6, -3)
  line L227 (-51.6, -3.8) -> (-51.6, -3)
  line L228 (-51.6, -3.8) -> (-51.6, -4.6)
  arc A91 (-55.2142, -7.8) -> (-54.5071, -7.5071) centre (-55.2142, -6.8) ccw
  line L229 (-54.5071, -7.5071) -> (-51.6, -4.6)
  arc A92 (-99.7929, 1.0071) -> (-99.5, 1.7142) centre (-100.5, 1.7142) ccw
  arc A93 (-107.5, 1.7142) -> (-107.2071, 1.0071) centre (-106.5, 1.7142) ccw
  line L230 (-99.7929, 1.0071) -> (-102.7, -1.9)
  line L231 (-107.2071, 1.0071) -> (-104.3, -1.9)
  line L232 (-103.5, -1.9) -> (-102.7, -1.9)
  line L233 (-103.5, -1.9) -> (-104.3, -1.9)
  line L234 (-107.5, 1.7142) -> (-107.5, 44.4858)
  line L235 (-99.5, 44.4858) -> (-99.5, 1.7142)
  arc A94 (-107.2071, 45.1929) -> (-107.5, 44.4858) centre (-106.5, 44.4858) ccw
  line L236 (-107.2071, 45.1929) -> (-104.3, 48.1)
  line L237 (-103.5, 48.1) -> (-104.3, 48.1)
  line L238 (-103.5, 48.1) -> (-102.7, 48.1)
  arc A95 (-99.5, 44.4858) -> (-99.7929, 45.1929) centre (-100.5, 44.4858) ccw
  line L239 (-99.7929, 45.1929) -> (-102.7, 48.1)
  arc A96 (-99.7929, -52.7929) -> (-99.5, -52.0858) centre (-100.5, -52.0858) ccw
  arc A97 (-107.5, -52.0858) -> (-107.2071, -52.7929) centre (-106.5, -52.0858) ccw
  line L240 (-99.7929, -52.7929) -> (-102.7, -55.7)
  line L241 (-107.2071, -52.7929) -> (-104.3, -55.7)
  line L242 (-103.5, -55.7) -> (-102.7, -55.7)
  line L243 (-103.5, -55.7) -> (-104.3, -55.7)
  line L244 (-107.5, -52.0858) -> (-107.5, -9.3142)
  line L245 (-99.5, -9.3142) -> (-99.5, -52.0858)
  arc A98 (-107.2071, -8.6071) -> (-107.5, -9.3142) centre (-106.5, -9.3142) ccw
  line L246 (-107.2071, -8.6071) -> (-104.3, -5.7)
  line L247 (-103.5, -5.7) -> (-104.3, -5.7)
  line L248 (-103.5, -5.7) -> (-102.7, -5.7)
  arc A99 (-99.5, -9.3142) -> (-99.7929, -8.6071) centre (-100.5, -9.3142) ccw
  line L249 (-99.7929, -8.6071) -> (-102.7, -5.7)
  arc A100 (-45.9929, 1.0071) -> (-45.7, 1.7142) centre (-46.7, 1.7142) ccw
  arc A101 (-53.7, 1.7142) -> (-53.4071, 1.0071) centre (-52.7, 1.7142) ccw
  line L250 (-45.9929, 1.0071) -> (-48.9, -1.9)
  line L251 (-53.4071, 1.0071) -> (-50.5, -1.9)
  line L252 (-49.7, -1.9) -> (-48.9, -1.9)
  line L253 (-49.7, -1.9) -> (-50.5, -1.9)
  line L254 (-53.7, 1.7142) -> (-53.7, 44.4858)
  line L255 (-45.7, 44.4858) -> (-45.7, 1.7142)
  arc A102 (-53.4071, 45.1929) -> (-53.7, 44.4858) centre (-52.7, 44.4858) ccw
  line L256 (-53.4071, 45.1929) -> (-50.5, 48.1)
  line L257 (-49.7, 48.1) -> (-50.5, 48.1)
  line L258 (-49.7, 48.1) -> (-48.9, 48.1)
  arc A103 (-45.7, 44.4858) -> (-45.9929, 45.1929) centre (-46.7, 44.4858) ccw
  line L259 (-45.9929, 45.1929) -> (-48.9, 48.1)
  arc A104 (-45.9929, -52.7929) -> (-45.7, -52.0858) centre (-46.7, -52.0858) ccw
  arc A105 (-53.7, -52.0858) -> (-53.4071, -52.7929) centre (-52.7, -52.0858) ccw
  line L260 (-45.9929, -52.7929) -> (-48.9, -55.7)
  line L261 (-53.4071, -52.7929) -> (-50.5, -55.7)
  line L262 (-49.7, -55.7) -> (-48.9, -55.7)
  line L263 (-49.7, -55.7) -> (-50.5, -55.7)
  line L264 (-53.7, -52.0858) -> (-53.7, -9.3142)
  line L265 (-45.7, -9.3142) -> (-45.7, -52.0858)
  arc A106 (-53.4071, -8.6071) -> (-53.7, -9.3142) centre (-52.7, -9.3142) ccw
  line L266 (-53.4071, -8.6071) -> (-50.5, -5.7)
  line L267 (-49.7, -5.7) -> (-50.5, -5.7)
  line L268 (-49.7, -5.7) -> (-48.9, -5.7)
  arc A107 (-45.7, -9.3142) -> (-45.9929, -8.6071) centre (-46.7, -9.3142) ccw
  line L269 (-45.9929, -8.6071) -> (-48.9, -5.7)
  arc A108 (-98.6929, -61.3071) -> (-97.9858, -61.6) centre (-97.9858, -60.6) ccw
  arc A109 (-97.9858, -53.6) -> (-98.6929, -53.8929) centre (-97.9858, -54.6) ccw
  line L270 (-98.6929, -61.3071) -> (-101.6, -58.4)
  line L271 (-98.6929, -53.8929) -> (-101.6, -56.8)
  line L272 (-101.6, -57.6) -> (-101.6, -58.4)
  line L273 (-101.6, -57.6) -> (-101.6, -56.8)
  line L274 (-97.9858, -53.6) -> (-55.2142, -53.6)
  line L275 (-55.2142, -61.6) -> (-97.9858, -61.6)
  arc A110 (-54.5071, -53.8929) -> (-55.2142, -53.6) centre (-55.2142, -54.6) ccw
  line L276 (-54.5071, -53.8929) -> (-51.6, -56.8)
  line L277 (-51.6, -57.6) -> (-51.6, -56.8)
  line L278 (-51.6, -57.6) -> (-51.6, -58.4)
  arc A111 (-55.2142, -61.6) -> (-54.5071, -61.3071) centre (-55.2142, -60.6) ccw
  line L279 (-54.5071, -61.3071) -> (-51.6, -58.4)
  arc A112 (-167.9929, 46.2929) -> (-167.2858, 46) centre (-167.2858, 47) ccw
  arc A113 (-167.2858, 54) -> (-167.9929, 53.7071) centre (-167.2858, 53) ccw
  line L280 (-167.9929, 46.2929) -> (-170.9, 49.2)
  line L281 (-167.9929, 53.7071) -> (-170.9, 50.8)
  line L282 (-170.9, 50) -> (-170.9, 49.2)
  line L283 (-170.9, 50) -> (-170.9, 50.8)
  line L284 (-167.2858, 54) -> (-124.5142, 54)
  line L285 (-124.5142, 46) -> (-167.2858, 46)
  arc A114 (-123.8071, 53.7071) -> (-124.5142, 54) centre (-124.5142, 53) ccw
  line L286 (-123.8071, 53.7071) -> (-120.9, 50.8)
  line L287 (-120.9, 50) -> (-120.9, 50.8)
  line L288 (-120.9, 50) -> (-120.9, 49.2)
  arc A115 (-124.5142, 46) -> (-123.8071, 46.2929) centre (-124.5142, 47) ccw
  line L289 (-123.8071, 46.2929) -> (-120.9, 49.2)
  arc A116 (-167.9929, -7.5071) -> (-167.2858, -7.8) centre (-167.2858, -6.8) ccw
  arc A117 (-167.2858, 0.2) -> (-167.9929, -0.0929) centre (-167.2858, -0.8) ccw
  line L290 (-167.9929, -7.5071) -> (-170.9, -4.6)
  line L291 (-167.9929, -0.0929) -> (-170.9, -3)
  line L292 (-170.9, -3.8) -> (-170.9, -4.6)
  line L293 (-170.9, -3.8) -> (-170.9, -3)
  line L294 (-167.2858, 0.2) -> (-124.5142, 0.2)
  line L295 (-124.5142, -7.8) -> (-167.2858, -7.8)
  arc A118 (-123.8071, -0.0929) -> (-124.5142, 0.2) centre (-124.5142, -0.8) ccw
  line L296 (-123.8071, -0.0929) -> (-120.9, -3)
  line L297 (-120.9, -3.8) -> (-120.9, -3)
  line L298 (-120.9, -3.8) -> (-120.9, -4.6)
  arc A119 (-124.5142, -7.8) -> (-123.8071, -7.5071) centre (-124.5142, -6.8) ccw
  line L299 (-123.8071, -7.5071) -> (-120.9, -4.6)
  arc A120 (-169.0929, 1.0071) -> (-168.8, 1.7142) centre (-169.8, 1.7142) ccw
  arc A121 (-176.8, 1.7142) -> (-176.5071, 1.0071) centre (-175.8, 1.7142) ccw
  line L300 (-169.0929, 1.0071) -> (-172, -1.9)
  line L301 (-176.5071, 1.0071) -> (-173.6, -1.9)
  line L302 (-172.8, -1.9) -> (-172, -1.9)
  line L303 (-172.8, -1.9) -> (-173.6, -1.9)
  line L304 (-176.8, 1.7142) -> (-176.8, 44.4858)
  line L305 (-168.8, 44.4858) -> (-168.8, 1.7142)
  arc A122 (-176.5071, 45.1929) -> (-176.8, 44.4858) centre (-175.8, 44.4858) ccw
  line L306 (-176.5071, 45.1929) -> (-173.6, 48.1)
  line L307 (-172.8, 48.1) -> (-173.6, 48.1)
  line L308 (-172.8, 48.1) -> (-172, 48.1)
  arc A123 (-168.8, 44.4858) -> (-169.0929, 45.1929) centre (-169.8, 44.4858) ccw
  line L309 (-169.0929, 45.1929) -> (-172, 48.1)
  arc A124 (-169.0929, -52.7929) -> (-168.8, -52.0858) centre (-169.8, -52.0858) ccw
  arc A125 (-176.8, -52.0858) -> (-176.5071, -52.7929) centre (-175.8, -52.0858) ccw
  line L310 (-169.0929, -52.7929) -> (-172, -55.7)
  line L311 (-176.5071, -52.7929) -> (-173.6, -55.7)
  line L312 (-172.8, -55.7) -> (-172, -55.7)
  line L313 (-172.8, -55.7) -> (-173.6, -55.7)
  line L314 (-176.8, -52.0858) -> (-176.8, -9.3142)
  line L315 (-168.8, -9.3142) -> (-168.8, -52.0858)
  arc A126 (-176.5071, -8.6071) -> (-176.8, -9.3142) centre (-175.8, -9.3142) ccw
  line L316 (-176.5071, -8.6071) -> (-173.6, -5.7)
  line L317 (-172.8, -5.7) -> (-173.6, -5.7)
  line L318 (-172.8, -5.7) -> (-172, -5.7)
  arc A127 (-168.8, -9.3142) -> (-169.0929, -8.6071) centre (-169.8, -9.3142) ccw
  line L319 (-169.0929, -8.6071) -> (-172, -5.7)
  arc A128 (-115.2929, 1.0071) -> (-115, 1.7142) centre (-116, 1.7142) ccw
  arc A129 (-123, 1.7142) -> (-122.7071, 1.0071) centre (-122, 1.7142) ccw
  line L320 (-115.2929, 1.0071) -> (-118.2, -1.9)
  line L321 (-122.7071, 1.0071) -> (-119.8, -1.9)
  line L322 (-119, -1.9) -> (-118.2, -1.9)
  line L323 (-119, -1.9) -> (-119.8, -1.9)
  line L324 (-123, 1.7142) -> (-123, 44.4858)
  line L325 (-115, 44.4858) -> (-115, 1.7142)
  arc A130 (-122.7071, 45.1929) -> (-123, 44.4858) centre (-122, 44.4858) ccw
  line L326 (-122.7071, 45.1929) -> (-119.8, 48.1)
  line L327 (-119, 48.1) -> (-119.8, 48.1)
  line L328 (-119, 48.1) -> (-118.2, 48.1)
  arc A131 (-115, 44.4858) -> (-115.2929, 45.1929) centre (-116, 44.4858) ccw
  line L329 (-115.2929, 45.1929) -> (-118.2, 48.1)
  arc A132 (-115.2929, -52.7929) -> (-115, -52.0858) centre (-116, -52.0858) ccw
  arc A133 (-123, -52.0858) -> (-122.7071, -52.7929) centre (-122, -52.0858) ccw
  line L330 (-115.2929, -52.7929) -> (-118.2, -55.7)
  line L331 (-122.7071, -52.7929) -> (-119.8, -55.7)
  line L332 (-119, -55.7) -> (-118.2, -55.7)
  line L333 (-119, -55.7) -> (-119.8, -55.7)
  line L334 (-123, -52.0858) -> (-123, -9.3142)
  line L335 (-115, -9.3142) -> (-115, -52.0858)
  arc A134 (-122.7071, -8.6071) -> (-123, -9.3142) centre (-122, -9.3142) ccw
  line L336 (-122.7071, -8.6071) -> (-119.8, -5.7)
  line L337 (-119, -5.7) -> (-119.8, -5.7)
  line L338 (-119, -5.7) -> (-118.2, -5.7)
  arc A135 (-115, -9.3142) -> (-115.2929, -8.6071) centre (-116, -9.3142) ccw
  line L339 (-115.2929, -8.6071) -> (-118.2, -5.7)
  arc A136 (-167.9929, -61.3071) -> (-167.2858, -61.6) centre (-167.2858, -60.6) ccw
  arc A137 (-167.2858, -53.6) -> (-167.9929, -53.8929) centre (-167.2858, -54.6) ccw
  line L340 (-167.9929, -61.3071) -> (-170.9, -58.4)
  line L341 (-167.9929, -53.8929) -> (-170.9, -56.8)
  line L342 (-170.9, -57.6) -> (-170.9, -58.4)
  line L343 (-170.9, -57.6) -> (-170.9, -56.8)
  line L344 (-167.2858, -53.6) -> (-124.5142, -53.6)
  line L345 (-124.5142, -61.6) -> (-167.2858, -61.6)
  arc A138 (-123.8071, -53.8929) -> (-124.5142, -53.6) centre (-124.5142, -54.6) ccw
  line L346 (-123.8071, -53.8929) -> (-120.9, -56.8)
  line L347 (-120.9, -57.6) -> (-120.9, -56.8)
  line L348 (-120.9, -57.6) -> (-120.9, -58.4)
  arc A139 (-124.5142, -61.6) -> (-123.8071, -61.3071) centre (-124.5142, -60.6) ccw
  line L349 (-123.8071, -61.3071) -> (-120.9, -58.4)
  arc A140 (-285.0929, 27.2929) -> (-284.3858, 27) centre (-284.3858, 28) ccw
  arc A141 (-284.3858, 35) -> (-285.0929, 34.7071) centre (-284.3858, 34) ccw
  line L350 (-285.0929, 27.2929) -> (-288, 30.2)
  line L351 (-285.0929, 34.7071) -> (-288, 31.8)
  line L352 (-288, 31) -> (-288, 30.2)
  line L353 (-288, 31) -> (-288, 31.8)
  line L354 (-284.3858, 35) -> (-241.6142, 35)
  line L355 (-241.6142, 27) -> (-284.3858, 27)
  arc A142 (-240.9071, 34.7071) -> (-241.6142, 35) centre (-241.6142, 34) ccw
  line L356 (-240.9071, 34.7071) -> (-238, 31.8)
  line L357 (-238, 31) -> (-238, 31.8)
  line L358 (-238, 31) -> (-238, 30.2)
  arc A143 (-241.6142, 27) -> (-240.9071, 27.2929) centre (-241.6142, 28) ccw
  line L359 (-240.9071, 27.2929) -> (-238, 30.2)
  arc A144 (216.0071, 46.2929) -> (216.7142, 46) centre (216.7142, 47) ccw
  arc A145 (216.7142, 54) -> (216.0071, 53.7071) centre (216.7142, 53) ccw
  line L360 (216.0071, 46.2929) -> (213.1, 49.2)
  line L361 (216.0071, 53.7071) -> (213.1, 50.8)
  line L362 (213.1, 50) -> (213.1, 49.2)
  line L363 (213.1, 50) -> (213.1, 50.8)
  line L364 (216.7142, 54) -> (259.4858, 54)
  line L365 (259.4858, 46) -> (216.7142, 46)
  arc A146 (260.1929, 53.7071) -> (259.4858, 54) centre (259.4858, 53) ccw
  line L366 (260.1929, 53.7071) -> (263.1, 50.8)
  line L367 (263.1, 50) -> (263.1, 50.8)
  line L368 (263.1, 50) -> (263.1, 49.2)
  arc A147 (259.4858, 46) -> (260.1929, 46.2929) centre (259.4858, 47) ccw
  line L369 (260.1929, 46.2929) -> (263.1, 49.2)
  arc A148 (216.0071, -7.5071) -> (216.7142, -7.8) centre (216.7142, -6.8) ccw
  arc A149 (216.7142, 0.2) -> (216.0071, -0.0929) centre (216.7142, -0.8) ccw
  line L370 (216.0071, -7.5071) -> (213.1, -4.6)
  line L371 (216.0071, -0.0929) -> (213.1, -3)
  line L372 (213.1, -3.8) -> (213.1, -4.6)
  line L373 (213.1, -3.8) -> (213.1, -3)
  line L374 (216.7142, 0.2) -> (259.4858, 0.2)
  line L375 (259.4858, -7.8) -> (216.7142, -7.8)
  arc A150 (260.1929, -0.0929) -> (259.4858, 0.2) centre (259.4858, -0.8) ccw
  line L376 (260.1929, -0.0929) -> (263.1, -3)
  line L377 (263.1, -3.8) -> (263.1, -3)
  line L378 (263.1, -3.8) -> (263.1, -4.6)
  arc A151 (259.4858, -7.8) -> (260.1929, -7.5071) centre (259.4858, -6.8) ccw
  line L379 (260.1929, -7.5071) -> (263.1, -4.6)
  arc A152 (214.9071, 1.0071) -> (215.2, 1.7142) centre (214.2, 1.7142) ccw
  arc A153 (207.2, 1.7142) -> (207.4929, 1.0071) centre (208.2, 1.7142) ccw
  line L380 (214.9071, 1.0071) -> (212, -1.9)
  line L381 (207.4929, 1.0071) -> (210.4, -1.9)
  line L382 (211.2, -1.9) -> (212, -1.9)
  line L383 (211.2, -1.9) -> (210.4, -1.9)
  line L384 (207.2, 1.7142) -> (207.2, 44.4858)
  line L385 (215.2, 44.4858) -> (215.2, 1.7142)
  arc A154 (207.4929, 45.1929) -> (207.2, 44.4858) centre (208.2, 44.4858) ccw
  line L386 (207.4929, 45.1929) -> (210.4, 48.1)
  line L387 (211.2, 48.1) -> (210.4, 48.1)
  line L388 (211.2, 48.1) -> (212, 48.1)
  arc A155 (215.2, 44.4858) -> (214.9071, 45.1929) centre (214.2, 44.4858) ccw
  line L389 (214.9071, 45.1929) -> (212, 48.1)
  arc A156 (214.9071, -52.7929) -> (215.2, -52.0858) centre (214.2, -52.0858) ccw
  arc A157 (207.2, -52.0858) -> (207.4929, -52.7929) centre (208.2, -52.0858) ccw
  line L390 (214.9071, -52.7929) -> (212, -55.7)
  line L391 (207.4929, -52.7929) -> (210.4, -55.7)
  line L392 (211.2, -55.7) -> (212, -55.7)
  line L393 (211.2, -55.7) -> (210.4, -55.7)
  line L394 (207.2, -52.0858) -> (207.2, -9.3142)
  line L395 (215.2, -9.3142) -> (215.2, -52.0858)
  arc A158 (207.4929, -8.6071) -> (207.2, -9.3142) centre (208.2, -9.3142) ccw
  line L396 (207.4929, -8.6071) -> (210.4, -5.7)
  line L397 (211.2, -5.7) -> (210.4, -5.7)
  line L398 (211.2, -5.7) -> (212, -5.7)
  arc A159 (215.2, -9.3142) -> (214.9071, -8.6071) centre (214.2, -9.3142) ccw
  line L399 (214.9071, -8.6071) -> (212, -5.7)
  arc A160 (268.7071, 1.0071) -> (269, 1.7142) centre (268, 1.7142) ccw
  arc A161 (261, 1.7142) -> (261.2929, 1.0071) centre (262, 1.7142) ccw
  line L400 (268.7071, 1.0071) -> (265.8, -1.9)
  line L401 (261.2929, 1.0071) -> (264.2, -1.9)
  line L402 (265, -1.9) -> (265.8, -1.9)
  line L403 (265, -1.9) -> (264.2, -1.9)
  line L404 (261, 1.7142) -> (261, 44.4858)
  line L405 (269, 44.4858) -> (269, 1.7142)
  arc A162 (261.2929, 45.1929) -> (261, 44.4858) centre (262, 44.4858) ccw
  line L406 (261.2929, 45.1929) -> (264.2, 48.1)
  line L407 (265, 48.1) -> (264.2, 48.1)
  line L408 (265, 48.1) -> (265.8, 48.1)
  arc A163 (269, 44.4858) -> (268.7071, 45.1929) centre (268, 44.4858) ccw
  line L409 (268.7071, 45.1929) -> (265.8, 48.1)
  arc A164 (268.7071, -52.7929) -> (269, -52.0858) centre (268, -52.0858) ccw
  arc A165 (261, -52.0858) -> (261.2929, -52.7929) centre (262, -52.0858) ccw
  line L410 (268.7071, -52.7929) -> (265.8, -55.7)
  line L411 (261.2929, -52.7929) -> (264.2, -55.7)
  line L412 (265, -55.7) -> (265.8, -55.7)
  line L413 (265, -55.7) -> (264.2, -55.7)
  line L414 (261, -52.0858) -> (261, -9.3142)
  line L415 (269, -9.3142) -> (269, -52.0858)
  arc A166 (261.2929, -8.6071) -> (261, -9.3142) centre (262, -9.3142) ccw
  line L416 (261.2929, -8.6071) -> (264.2, -5.7)
  line L417 (265, -5.7) -> (264.2, -5.7)
  line L418 (265, -5.7) -> (265.8, -5.7)
  arc A167 (269, -9.3142) -> (268.7071, -8.6071) centre (268, -9.3142) ccw
  line L419 (268.7071, -8.6071) -> (265.8, -5.7)
  arc A168 (216.0071, -61.3071) -> (216.7142, -61.6) centre (216.7142, -60.6) ccw
  arc A169 (216.7142, -53.6) -> (216.0071, -53.8929) centre (216.7142, -54.6) ccw
  line L420 (216.0071, -61.3071) -> (213.1, -58.4)
  line L421 (216.0071, -53.8929) -> (213.1, -56.8)
  line L422 (213.1, -57.6) -> (213.1, -58.4)
  line L423 (213.1, -57.6) -> (213.1, -56.8)
  line L424 (216.7142, -53.6) -> (259.4858, -53.6)
  line L425 (259.4858, -61.6) -> (216.7142, -61.6)
  arc A170 (260.1929, -53.8929) -> (259.4858, -53.6) centre (259.4858, -54.6) ccw
  line L426 (260.1929, -53.8929) -> (263.1, -56.8)